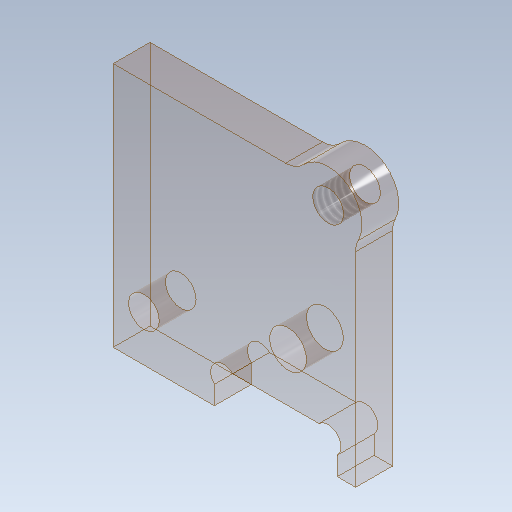
# Autodesk Inventor part: カウンター展開支柱test
Saved by Autodesk Inventor 2020.2 (Build 242310000, 310)
## iProperties
Created: 2020-04-03
Part Number: カウンター展開支柱test
Material: ポリカーボネート、スモーク
Document SubType Name: Modeling
Designer: aoyama
Density: 1.2 g/cm^3
Appearance: ポリカーボネート - スモーク
Mass: 1.27117 g
Surface Area: 10.44 cm^2
Volume: 1.05931 cm^3
Author: aoyama
Autodesk Inventor part; units mm, degrees
ref_plane "YZ Plane" through (0, 0, 0) normal (1, 0, 0) x (0, 1, 0)
ref_plane "XZ Plane" through (0, 0, 0) normal (0, 1, 0) x (-1, 0, 0)
ref_plane "XY Plane" through (0, 0, 0) normal (0, 0, 1) x (1, 0, 0)
sketch "スケッチ1" plane through (0, 0, 0) normal (0, 0, 1) x (1, 0, 0)
  line L0 (0, 0) -> (0, 15) construction
  line L1 (2.5, 0) -> (2.5, 15)
  line L2 (-2.5, 15) -> (-2.5, 0)
  arc A0 (-2.5, 0) -> (2.5, 0) centre (0, 0) ccw
  arc A1 (2.5, 15) -> (-2.5, 15) centre (0, 15) ccw
  circle A2 centre (0, 15) radius 1.5
  circle A3 centre (0, 0) radius 1.5
  line L3 (-2.5, 17.5) -> (2.5, 17.5)
  line L4 (2.5, 17.5) -> (2.5, -2.5)
  line L5 (2.5, -2.5) -> (-2.5, -2.5)
  line L6 (-2.5, -2.5) -> (-2.5, 17.5)
  line L7 (0, 12.5) -> (15, 12.5)
  line L8 (17.5, 12.5) -> (-2.5, 12.5)
  line L9 (17.5, 17.5) -> (17.5, 12.5)
  line L10 (-2.5, 17.5) -> (17.5, 17.5)
  arc A4 (15, 12.5) -> (15, 17.5) centre (15, 15) ccw
  circle A5 centre (15, 15) radius 1.5
  line L11 (-2.5, 17.5) -> (17.2387, 17.5)
  line L12 (17.2387, 17.5) -> (17.2387, -2.5)
  line L13 (17.2387, -2.5) -> (-2.5, -2.5)
  line L14 (-2.5, -2.5) -> (-2.5, 17.5)
  line L15 (15.7387, -2.5) -> (5.7387, -2.5)
  line L16 (5.7387, -2.5) -> (5.7387, 0.5)
  line L17 (5.7387, 0.5) -> (15.7387, 0.5)
  line L18 (15.7387, 0.5) -> (15.7387, -2.5)
  circle A6 centre (11.7387, 4.5) radius 1.5
  circle A7 centre (0, 0) radius 1.25
  circle A8 centre (15, 15) radius 1.25 construction
  circle A9 centre (0, 1.25) radius 1.25
  circle A10 centre (15, 16.25) radius 1.25
  line L19 (15, 16.25) -> (15, 15)
  circle A11 centre (15, 16.25) radius 2.75
  circle A12 centre (6.4812, -0.2425) radius 1.05
  circle A13 centre (14.9962, -0.2425) radius 1.05
  line L20 (14.9962, -0.2425) -> (15.7387, 0.5)
  line L21 (5.7387, 0.5) -> (6.4812, -0.2425)
  line L22 (15, 15) -> (0, 15)
  point P0 (0, 7.5)
  point P1 (0, -2.5)
  point P2 (2.5, 0)
  point P3 (0, 17.5)
  point P4 (2.5, 15)
  point P5 (2.5, 15)
  point P6 (2.5, 0)
  point P7 (2.5, -2.5)
  point P8 (17.5, 12.5)
  point P9 (17.2387, 12.5)
  point P10 (2.5, 12.5)
  point P11 (-2.5, 12.5)
  point P12 (15, 15.625)
  point P13 (17.4495, 17.5)
  point P14 (12.5505, 17.5)
  point P15 (5.7387, -0.9849)
  point P16 (7.2236, 0.5)
  point P17 (14.2538, 0.5)
  point P18 (15.7387, -0.9849)
  point P19 (16.5612, 17.5)
  point P20 (12.5505, 17.5)
  point P21 (17.2387, 14.6529)
  point P22 (0, 17.5)
  dimension "d28" = 2.1
  dimension "d29" = 2.1
  dimension "d0" = 5
  dimension "d1" = 15
  dimension "d2" = 3
  dimension "d3" = 3
  dimension "d8" = 90
  dimension "d10" = 10
  dimension "d11" = 3
  dimension "d12" = 1.5
  dimension "d13" = 3
  dimension "d14" = 4
  dimension "d15" = 4
  dimension "d16" = 2.5
  dimension "d17" = 2.5
  dimension "d22" = 2.5
  dimension "d23" = 1.25
  dimension "d24" = 2.5
  dimension "d25" = 1.25
  dimension "d26" = 5.5
  dimension "d30" = 45
  dimension "d31" = 45
  dimension "d32" = 11.7387
  constraints: 48 end point, 12 centre point, 6 coincident, 6 point on circle, 4 tangent, 2 midpoint, 2 point on line, 2 vertical, 1 parallel, 23 other
  measures "d0" diameter of A1
  measures "d1" distance of L0.end L0.start
  measures "d2" diameter of A2
  measures "d3" diameter of A3
  measures "d10" distance between parallel lines of L18 L16
  measures "d11" distance of L17.end L15.start
  measures "d12" distance between parallel lines of L12 L18
  measures "d13" diameter of A6
  measures "d14" distance from line of A6.centre L17
  measures "d15" distance from line of A6.centre L18
  measures "d16" diameter of A7
  measures "d17" diameter of A8
  measures "d22" diameter of A9
  measures "d23" distance of L0.start A9.centre
  measures "d24" diameter of A10
  measures "d25" distance of L19.start L19.end
  measures "d26" diameter of A11
  measures "d30" angle of L17 L21
  measures "d31" angle of L17 L20
  measures "d32" distance from line of A6.centre L0
extrude "押し出し1" add sketch "スケッチ1" along normal blind 3 contours A0 L2 L8 L7 L1 | L4 L5 A0 | L1 L7 L8 L12 L13 L18 A13 L17 A12 L16 L4 | A2 | L7 L8 L2 A1 L1 | L1 L22 A11 L12 A4 L7 | L5 L6 A0 | A1 L3 L4 | L4 L10 A11 L22 | A4 L12 L8 | A1 L6 L3 | L22 A5 A11 | A11 L10 A10 A5 L22 | A11 L10 | A5 L22 A10 | A5 A10 A4 L12 A11 | A5 A10 L22 | A4 L12 L10 A11 L9 | A11 L12 A4 | L9 A11 | L10 L12 A4 | A3 A9 A7 | A7 A9 picked at (17.2844, 15.5147) picked at (1.4027, -0.1172) picked at (-0.0628, -0.8242)
thread "ねじ1" size "M3x0.5" class "6H" standard "ANSI Metric M Profile" full length
fillet "フィレット1" radius 2 2 edges at (12.5505, 17.5, 1.5) (17.2387, 14.6529, 1.5)
sketch "スケッチ2" plane through (0, 0, 3) normal (0, 0, 1) x (1, 0, 0)
  line L0 (-2.5, 17.5) -> (-2.5, -2.5) projected
  line L1 (-2.5, -2.5) -> (5.7387, -2.5) projected
  line L2 (5.7387, -2.5) -> (5.7387, -0.9849) projected
  arc A0 (7.2236, 0.5) -> (5.7387, -0.9849) centre (6.4812, -0.2425) ccw projected
  line L3 (7.2236, 0.5) -> (14.2538, 0.5) projected
  arc A1 (15.7387, -0.9849) -> (14.2538, 0.5) centre (14.9962, -0.2425) ccw projected
  line L4 (15.7387, -0.9849) -> (15.7387, -2.5) projected
  line L5 (15.7387, -2.5) -> (17.2387, -2.5) projected
  line L6 (17.2387, -2.5) -> (17.2387, 14.1062) projected
  arc A2 (17.454, 15.0089) -> (17.2387, 14.1062) centre (19.2387, 14.1062) ccw projected
  arc A3 (17.454, 15.0089) -> (12.9945, 18.1316) centre (15, 16.25) ccw projected
  arc A4 (11.5359, 17.5) -> (12.9945, 18.1316) centre (11.5359, 19.5) ccw projected
  line L7 (11.5359, 17.5) -> (-2.5, 17.5) projected
  circle A5 centre (15, 16.25) radius 1.25 projected
  circle A6 centre (11.7387, 4.5) radius 1.5 projected
  circle A7 centre (0, 1.25) radius 1.25 projected
  point P0 (0, 0)
